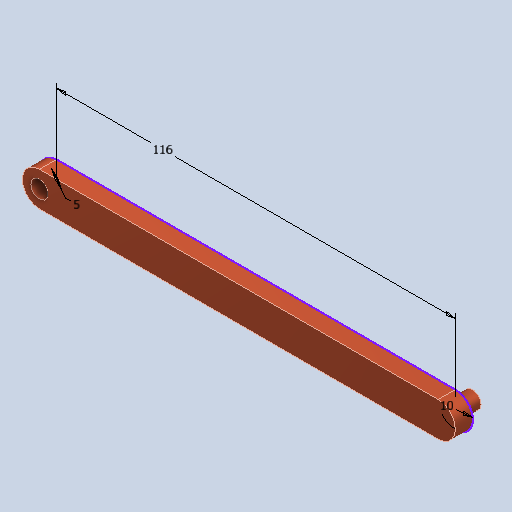
# Autodesk Inventor part: Part1
Saved by Autodesk Inventor 2022 (Build 260153000, 153)
## iProperties
Created: 2022-03-14
Part Number: Part1
Material: Copper, Alloy
Document SubType Name: Modeling
Designer: br4ch
Density: 8.92 g/cm^3
Appearance: Copper - Satin
Mass: 55.2389 g
Surface Area: 39.1197 cm^2
Volume: 6.1927 cm^3
Author: br4ch
Autodesk Inventor part; units mm, degrees
ref_plane "YZ Plane" through (0, 0, 0) normal (1, 0, 0) x (0, 1, 0)
ref_plane "XZ Plane" through (0, 0, 0) normal (0, 1, 0) x (-1, 0, 0)
ref_plane "XY Plane" through (0, 0, 0) normal (0, 0, 1) x (1, 0, 0)
sketch "Sketch1" plane through (0, 0, 0) normal (0, 0, 1) x (1, 0, 0)
  line L0 (-20, 3) -> (96, 3) construction
  line L1 (-20, -2) -> (96, -2)
  line L2 (96, 8) -> (-20, 8)
  arc A0 (-20, 8) -> (-20, -2) centre (-20, 3) ccw
  arc A1 (96, -2) -> (96, 8) centre (96, 3) ccw
  circle A2 centre (-20, 3) radius 2.5
  circle A3 centre (96, 3) radius 2.5
  point P0 (0, 0)
  point P1 (38, 3)
  dimension "d0" = 10
  dimension "d1" = 5
  dimension "d2" = 116
  constraints: 8 end point, 4 centre point, 4 point on circle, 4 tangent, 2 coincident, 1 equal radius, 1 horizontal, 1 midpoint, 1 parallel
  measures "d0" diameter of A1
  measures "d1" diameter of A2
  measures "d2" distance of L0.end L0.start
extrude "Extrusion1" add sketch "Sketch1" along normal blind 5 contours A0 L2 A1 L1 | A3
extrude "Extrusion2" add sketch "Sketch1" against normal blind 5 contours A3
body "Solid1"
